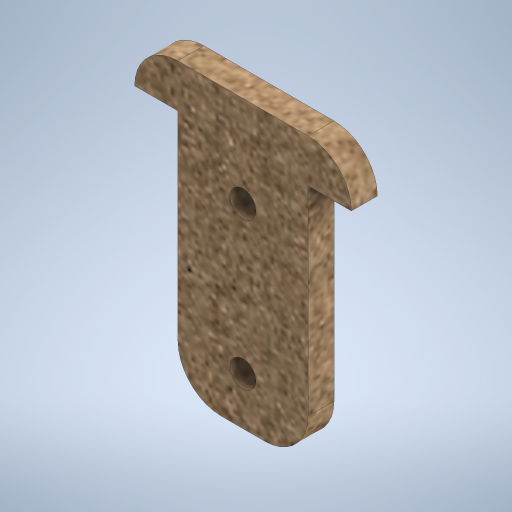
# Autodesk Inventor part: Motor_Support
Saved by Autodesk Inventor 2024 (Build 280153000, 153)
## iProperties
Created: 2023-11-23
Part Number: Motor_Support
Material: MDF Tablero de fibras de densidad media
Document SubType Name: Modeling
Designer: marco
Density: 0.8 g/cm^3
Appearance: Cartón - Ondulado
Author: marco
Autodesk Inventor part; units mm, degrees
ref_plane "YZ Plane" through (0, 0, 0) normal (1, 0, 0) x (0, 1, 0)
ref_plane "XZ Plane" through (0, 0, 0) normal (0, 1, 0) x (-1, 0, 0)
ref_plane "XY Plane" through (0, 0, 0) normal (0, 0, 1) x (1, 0, 0)
sketch "Boceto1" plane through (0, 0, 0) normal (0, 0, 1) x (1, 0, 0)
  point P0 (0, 0)
sketch "Boceto2" plane through (0, 0, 0) normal (0, 0, 1) x (1, 0, 0)
  line L0 (-12.5, 11.5) -> (-7.5, 11.5)
  circle A0 centre (0, 6) radius 1.5
  circle A1 centre (0, -11) radius 1.5
  line L1 (7.5, 11.5) -> (12.5, 11.5)
  arc A2 (12.5, 11.5) -> (7.5, 16.5) centre (7.5, 11.5) ccw
  line L2 (7.5, 16.5) -> (-7.5, 16.5)
  arc A3 (-7.5, 16.5) -> (-12.5, 11.5) centre (-7.5, 11.5) ccw
  line L3 (-7.5, 11.5) -> (-7.5, -11.5)
  arc A4 (-7.5, -11.5) -> (-2.5, -16.5) centre (-2.5, -11.5) ccw
  line L4 (-2.5, -16.5) -> (2.5, -16.5)
  arc A5 (2.5, -16.5) -> (7.5, -11.5) centre (2.5, -11.5) ccw
  line L5 (7.5, -11.5) -> (7.5, 11.5)
  point P0 (0, 0)
  point P1 (-2.5, -16.5)
  point P2 (7.5, -11.5)
  constraints: 12 end point, 8 point on circle, 6 centre point
extrude "Extrusión1" add sketch "Boceto2" along normal blind 3
